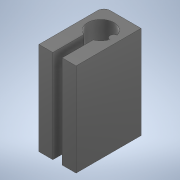
# Autodesk Inventor part: YsupportA
Saved by Autodesk Inventor 2020.2 (Build 242310000, 310)
## iProperties
Created: 2020-08-09
Part Number: YsupportA
Material: Generic
Document SubType Name: Modeling
Designer: JK
Density: 1 g/cm^3
Appearance: Smooth - Black
Author: JK
Autodesk Inventor part; units mm, degrees
ref_plane "YZ Plane" through (0, 0, 0) normal (1, 0, 0) x (0, 1, 0)
ref_plane "XZ Plane" through (0, 0, 0) normal (0, 1, 0) x (-1, 0, 0)
ref_plane "XY Plane" through (0, 0, 0) normal (0, 0, 1) x (1, 0, 0)
sketch "Sketch1" plane through (0, 0, 0) normal (0, 1, 0) x (-1, 0, 0)
  circle A0 centre (0, 0) radius 4.25
  line L0 (6, 7) -> (-6, 7)
  line L1 (-6, 7) -> (-6, -7)
  line L2 (-6, -7) -> (6, -7)
  line L3 (6, -7) -> (6, 7)
  line L4 (6, 7) -> (-6, 7)
  line L5 (-6, 7) -> (-6, 14)
  line L6 (-6, 14) -> (6, 14)
  line L7 (6, 14) -> (6, 7)
  point P0 (-6, 7)
  dimension "d0" = 8.5
  dimension "d1" = 6
  dimension "d2" = 14
  dimension "d3" = 12
  dimension "d4" = 7
  dimension "d5" = 7
  constraints: 16 end point, 4 parallel, 2 horizontal, 2 perpendicular, 1 centre point, 1 coincident
  measures "d0" diameter of A0
  measures "d1" distance from line of L1 point (0, 0)
  measures "d2" distance of L0.end L1.end
  measures "d3" distance between parallel lines of L1 L3
  measures "d4" distance from line of point (0, 0) L2
  measures "d5" distance of L6.end L0.start
extrude "Extrusion1" add sketch "Sketch1" along normal blind 35
sketch "Sketch2" plane through (0, 35, 0) normal (0, 1, 0) x (1, 0, 0)
  line L0 (-1.5, -16.1218) -> (1.5, -16.1218)
  line L1 (1.5, -16.1218) -> (1.5, -1.7668)
  line L2 (1.5, -1.7668) -> (-1.5, -1.7668)
  line L3 (-1.5, -1.7668) -> (-1.5, -16.1218)
  point P0 (0, 0)
  dimension "d8" = 1.5
  dimension "d9" = 1.5
  constraints: 8 end point, 2 parallel, 1 horizontal, 1 perpendicular
  measures "d8" distance from line of point (0, 0) L3
  measures "d9" distance from line of point (0, 0) L1
extrude "Extrusion2" cut sketch "Sketch2" against normal through all
sketch "Sketch3" plane through (-6, 0, -7) normal (-1, 0, 0) x (0, 0, 1)
  circle A0 centre (15, 15) radius 2.75
  line L0 (21, 0) -> (21, 35) projected
  line L1 (0, 0) -> (21, 0) projected
  point P0 (7, 0)
  dimension "d12" = 5.5
  dimension "d13" = 6
  dimension "d14" = 15
  constraints: 1 centre point
  measures "d12" diameter of A0
  measures "d13" distance from line of L0 A0.centre
  measures "d14" distance from line of L1 A0.centre
extrude "Extrusion3" cut sketch "Sketch3" against normal blind 10
sketch "Sketch4" plane through (0, 35, 0) normal (0, 1, 0) x (1, 0, 0)
  arc A0 (1.5, -3.9765) -> (-1.5, -3.9765) centre (0, 0) ccw projected
  circle A1 centre (4.25, 0) radius 1.25
  point P0 (4.0662, 1.2364)
  point P1 (4.0662, -1.2364)
  dimension "d17" = 2.5
  constraints: 1 centre point, 1 point on circle
  measures "d17" diameter of A1
extrude "Extrusion4" add sketch "Sketch4" against normal blind 14.5 contours A1 A0 picked at (3.8196, 0)
sketch "Sketch5" plane through (0, 35, 0) normal (0, 1, 0) x (1, 0, 0)
  line L0 (1.5, -14) -> (6, -14) projected
  line L1 (6, -14) -> (36, -14)
  line L2 (36, -14) -> (36, 7)
  line L3 (36, 7) -> (6, 7)
  line L4 (6, 7) -> (6, -14)
  circle A0 centre (21, -3.5) radius 2.75
  point P0 (0, 0)
  dimension "d20" = 30
  dimension "d21" = 15
  dimension "d22" = 10.5
  dimension "d23" = 5.5
  constraints: 8 end point, 2 parallel, 1 centre point, 1 horizontal, 1 perpendicular
  measures "d20" distance between parallel lines of L4 L2
  measures "d21" distance from line of L4 A0.centre
  measures "d22" distance from line of L1 A0.centre
  measures "d23" diameter of A0
extrude "Extrusion5" add sketch "Sketch5" against normal blind 5
sketch "Sketch6" plane through (0, 35, 0) normal (0, 1, 0) x (1, 0, 0)
  circle A0 centre (21, -3.5) radius 2.75 projected
  circle A1 centre (21, -3.5) radius 4.75
  point P0 (0, 0)
  dimension "d26" = 9.5
  constraints: 1 centre point, 1 coincident
  measures "d26" diameter of A1
extrude "Extrusion6" cut sketch "Sketch6" against normal blind 2
sketch "Sketch7" plane through (-6, 0, -7) normal (-1, 0, 0) x (0, 0, 1)
  circle A0 centre (15, 15) radius 2.75 projected
  circle A1 centre (15, 15) radius 4.75
  point P0 (7, 0)
  dimension "d29" = 9.5
  constraints: 1 centre point, 1 coincident
  measures "d29" diameter of A1
extrude "Extrusion7" cut sketch "Sketch7" against normal blind 2
fillet "Fillet1" radius 2 3 edges at (-6, 17.5, -7) (36, 32.5, -7) (36, 32.5, 14)
sketch "Sketch9" plane through (0, 35, 0) normal (0, 1, 0) x (1, 0, 0)
  line L0 (-21.5057, -29.1514) -> (41.8439, -29.1514)
  line L1 (41.8439, -29.1514) -> (41.8439, 16.5719)
  line L2 (41.8439, 16.5719) -> (-21.5057, 16.5719)
  line L3 (-21.5057, 16.5719) -> (-21.5057, -29.1514)
  point P0 (0, 0)
  constraints: 8 end point, 2 parallel, 1 horizontal, 1 perpendicular
extrude "Extrusion8" cut sketch "Sketch9" against normal blind 5
body "Solid1"
